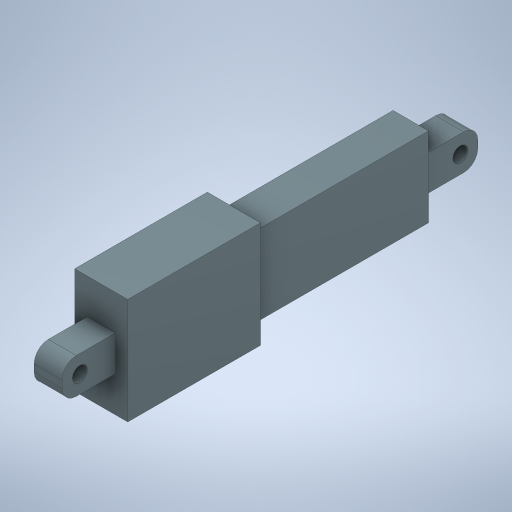
# Autodesk Inventor part: 각도조절 액추에이터_최소
Saved by Autodesk Inventor 2024 (Build 280153000, 153)
## iProperties
Created: 2024-04-05
Part Number: 각도조절 액추에이터_최소
Material: 납
Document SubType Name: Modeling
Designer: kkamin5
Density: 11.34 g/cm^3
Appearance: 납
Author: kkamin5
Autodesk Inventor part; units mm, degrees
ref_plane "YZ Plane" through (0, 0, 0) normal (1, 0, 0) x (0, 1, 0)
ref_plane "XZ Plane" through (0, 0, 0) normal (0, 1, 0) x (-1, 0, 0)
sketch "스케치1" plane through (0, 0, 0) normal (0, 0, 1) x (1, 0, 0)
  line L0 (-7.5, -15) -> (7.5, -15)
  line L1 (7.5, -15) -> (7.5, 15)
  line L2 (7.5, 15) -> (-7.5, 15)
  line L3 (-7.5, 15) -> (-7.5, -15)
  point P0 (0, 0)
  dimension "d0" = 15
  dimension "d1" = 30
  dimension "d2" = 15
  dimension "d3" = 7.5
  constraints: 8 end point, 2 parallel, 1 horizontal, 1 perpendicular
  measures "d0" distance of L1.end L2.end
  measures "d1" distance of L0.end L1.end
  measures "d2" distance from line of point (0, 0) L2
  measures "d3" distance from line of point (0, 0) L1
extrude "돌출1" add sketch "스케치1" against normal blind 37.5
sketch "스케치2" plane through (0, 0, -37.5) normal (0, 0, -1) x (-1, 0, 0)
  line L0 (5, 11.25) -> (-5, 11.25)
  line L1 (-5, 11.25) -> (-5, -11.25)
  line L2 (-5, -11.25) -> (5, -11.25)
  line L3 (5, -11.25) -> (5, 11.25)
  line L4 (5, 11.25) -> (-5, -11.25) construction
  line L5 (-5, 11.25) -> (5, -11.25) construction
  line L6 (-4, -10) -> (4, -10)
  line L7 (4, -10) -> (4, 10)
  line L8 (4, 10) -> (-4, 10)
  line L9 (-4, 10) -> (-4, -10)
  line L10 (-4, -10) -> (4, 10) construction
  line L11 (4, -10) -> (-4, 10) construction
  point P0 (0, 0)
  dimension "d6" = 10
  dimension "d7" = 22.5
  dimension "d10" = 8
  dimension "d11" = 20
  constraints: 24 end point, 4 midpoint, 4 parallel, 2 horizontal, 2 perpendicular
  measures "d6" distance of L2.end L1.end
  measures "d7" distance of L1.end L0.end
  measures "d10" distance of L8.end L7.end
  measures "d11" distance of L7.end L6.end
extrude "돌출2" add sketch "스케치2" along normal blind 50
sketch "스케치3" plane through (0, 0, 0) normal (0, 0, 1) x (1, 0, 0)
  line L0 (-3.95, -5) -> (3.95, -5)
  line L1 (3.95, -5) -> (3.95, 5)
  line L2 (3.95, 5) -> (-3.95, 5)
  line L3 (-3.95, 5) -> (-3.95, -5)
  line L4 (-3.95, -5) -> (3.95, 5) construction
  line L5 (3.95, -5) -> (-3.95, 5) construction
  point P0 (0, 0)
  dimension "d12" = 7.9
  dimension "d13" = 10
  constraints: 12 end point, 2 midpoint, 2 parallel, 1 horizontal, 1 perpendicular
  measures "d12" distance of L2.end L1.end
  measures "d13" distance of L1.end L0.end
extrude "돌출3" add sketch "스케치3" along normal blind 15
sketch "스케치4" plane through (3.95, -5, 0) normal (1, 0, 0) x (0, 0, -1)
  circle A0 centre (-10, 5) radius 2.1
  line L0 (0, 0) -> (-15, 0) projected
  line L1 (-15, 0) -> (-15, 10) projected
  point P0 (0, 5)
  dimension "d16" = 4.2
  dimension "d17" = 5
  dimension "d18" = 5
  constraints: 1 centre point
  measures "d16" diameter of A0
  measures "d17" distance from line of L0 A0.centre
  measures "d18" distance from line of L1 A0.centre
extrude "돌출4" cut sketch "스케치4" against normal blind 15
sketch "스케치5" plane through (0, 0, -87.5) normal (0, 0, -1) x (-1, 0, 0)
  line L0 (-5, 11.25) -> (5, 11.25) projected
  line L1 (5, -11.25) -> (-5, -11.25) projected
  line L2 (5, 11.25) -> (-5, 11.25)
  line L3 (-5, 11.25) -> (-5, -11.25)
  line L4 (-5, -11.25) -> (5, -11.25)
  line L5 (5, -11.25) -> (5, 11.25)
  point P0 (7.5, 15)
  point P1 (-7.5, -15)
  constraints: 8 end point, 2 parallel, 1 horizontal, 1 perpendicular
extrude "돌출5" add sketch "스케치5" against normal blind 2
ref_plane "작업 평면1" through (0, 0, -43.75) normal (0, 0, 1) x (1, 0, 0)
mirror "미러1" about plane through (0, 0, -43.75) normal (0, 0, 1) of "돌출3"
mirror "미러2" about plane through (0, 0, -43.75) normal (0, 0, 1) of "돌출4"
fillet "모깎기1" radius 4 4 edges at (0, -5, 15) (0, 5, 15) (0, -5, -102.5) (0, 5, -102.5)
